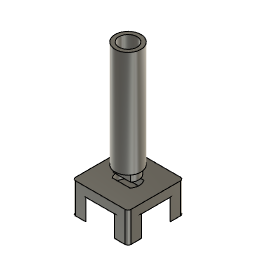
rotating arm cube v4 (Autodesk Fusion 360 design; units mm, degrees)
Autodesk Fusion 360 part; units mm, degrees
note: some values were not read from the file. Set by a fixed rule: which sketch regions a step uses.
sketch "Sketch1" plane through (0, 0, 0) normal (0, 0, 1) x (1, 0, 0)
  line L0 (0, 0) -> (18.3, 0)
  line L1 (18.3, 0) -> (18.3, -18.3)
  line L2 (18.3, -18.3) -> (0, -18.3)
  line L3 (0, -18.3) -> (0, 0)
  circle A0 centre (9.15, -9.15) radius 10.675
  dimension "d1" = 18.3
  dimension "d2" = 18.3
  dimension "d3" = 21.35
  constraint horizontal L0
  constraint vertical L1
  constraint horizontal L2
  constraint vertical L3
  constraint coincident L0.start L3.end
  measures "d1" distance of L0.start L0.end
  measures "d2" distance of L0.start L2.end
  measures "d3" diameter of A0
extrude "Extrude1" add sketch "Sketch1" along normal blind 10 contours L0 L3 A0 | L0 L1 L2 L3 A0 | L0 L1 A0 | L2 L3 A0 | L1 L2 A0 makes body 1
fillet "Fillet1" radius 5.5 4 edges at (18.3, -18.3, 5) (0, -18.3, 5) (18.3, 0, 5) (0, 0, 5) on bodies 1
extrude "Extrude2" add sketch "Sketch1" along normal blind 3 from surface at 10 separate body contours L0 L3 A0 | L0 L1 L2 L3 A0 | L0 L1 A0 | L2 L3 A0 | L1 L2 A0 makes body 2
sketch "Sketch2" plane through (0, 0, 10) normal (0, 0, 1) x (-1, 0, 0)
  arc A0 (-5.5, 0) -> (0, 5.5) centre (-5.5, 5.5) ccw
  line L0 (0, 5.5) -> (0, 12.8)
  arc A1 (0, 12.8) -> (-5.5, 18.3) centre (-5.5, 12.8) ccw
  line L1 (-5.5, 18.3) -> (-12.8, 18.3)
  arc A2 (-12.8, 18.3) -> (-18.3, 12.8) centre (-12.8, 12.8) ccw
  line L2 (-18.3, 12.8) -> (-18.3, 5.5)
  arc A3 (-18.3, 5.5) -> (-12.8, 0) centre (-12.8, 5.5) ccw
  line L3 (-12.8, 0) -> (-5.5, 0)
  line L4 (0, 0) -> (-18.3, 0)
  line L5 (-18.3, 0) -> (-18.3, 18.3)
  line L6 (-18.3, 18.3) -> (0, 18.3)
  line L7 (0, 18.3) -> (0, 0)
  constraint horizontal L4
  constraint vertical L5
  constraint horizontal L6
  constraint vertical L7
  constraint coincident L4.start L7.end
extrude "Extrude3" add sketch "Sketch2" against normal blind 7 contours A0 L4 L7 | A3 L4 L5 | A1 L6 L7 | A2 L5 L6 bodies 2
fillet "Fillet2" radius 1 4 edges at (0, -18.3, 8) (18.3, -18.3, 8) (18.3, 0, 8) (0, 0, 8) on bodies 2
sketch "Sketch3" plane through (0, 0, 13) normal (0, 0, 1) x (-1, 0, 0)
  arc A0 (-1, 0) -> (0, 1) centre (-1, 1) ccw
  line L0 (0, 1) -> (0, 17.3)
  arc A1 (0, 17.3) -> (-1, 18.3) centre (-1, 17.3) ccw
  line L1 (-1, 18.3) -> (-17.3, 18.3)
  arc A2 (-17.3, 18.3) -> (-18.3, 17.3) centre (-17.3, 17.3) ccw
  line L2 (-18.3, 17.3) -> (-18.3, 1)
  arc A3 (-18.3, 1) -> (-17.3, 0) centre (-17.3, 1) ccw
  line L3 (-17.3, 0) -> (-1, 0)
  line L4 (-9.15, 0) -> (-9.15, 18.3) construction
  line L5 (0, 9.15) -> (-18.3, 9.15) construction
  circle A4 centre (-9.15, 9.15) radius 3.5
  line L6 (-8.15, 14.15) -> (-10.15, 14.15)
  line L7 (-10.15, 14.15) -> (-10.15, 4.15)
  line L8 (-10.15, 4.15) -> (-8.15, 4.15)
  line L9 (-8.15, 4.15) -> (-8.15, 14.15)
  line L10 (-8.15, 14.15) -> (-10.15, 4.15) construction
  line L11 (-10.15, 14.15) -> (-8.15, 4.15) construction
  line L12 (-8.05, 4.05) -> (-10.25, 4.05)
  line L13 (-10.25, 4.05) -> (-10.25, 14.25)
  line L14 (-10.25, 14.25) -> (-8.05, 14.25)
  line L15 (-8.05, 14.25) -> (-8.05, 4.05)
  line L16 (-8.05, 4.05) -> (-10.25, 14.25) construction
  line L17 (-10.25, 4.05) -> (-8.05, 14.25) construction
  circle A5 centre (-9.15, 9.15) radius 3.6
  point P0 (-9.15, 9.15)
  point P1 (-9.15, 9.15)
  dimension "d15" = 7
  dimension "d16" = 2
  dimension "d17" = 10
  dimension "d18" = 2.2
  dimension "d19" = 10.2
  dimension "d20" = 7.2
  constraint midpoint L3 L4.start
  constraint midpoint L1 L4.end
  constraint midpoint L0 L5.start
  constraint midpoint L2 L5.end
  constraint midpoint L5 P1
  constraint horizontal L6
  constraint perpendicular L6 L7
  constraint parallel L6 L8
  constraint parallel L7 L9
  constraint coincident L10 P1
  constraint coincident L11 P1
  constraint coincident P1 P0
  constraint horizontal L12
  constraint perpendicular L12 L13
  constraint parallel L12 L14
  constraint parallel L13 L15
  constraint coincident L16 P1
  constraint coincident L17 P1
  measures "d15" diameter of A4
  measures "d16" distance of L7.end L8.end
  measures "d17" distance of L6.end L7.end
  measures "d18" distance of L13.end L14.end
  measures "d19" distance of L12.end L13.end
  measures "d20" diameter of A5
extrude "Extrude5" add sketch "Sketch3" against normal blind 2.5 separate body contours A4 L15 | A4 L9 L15 | A4 L7 L9 | A4 L7 L13 | A4 L13 makes body 3
extrude "Extrude6" add sketch "Sketch3" along normal blind 10 contours A4 L15 | A4 L9 L15 | A4 L7 L9 | A4 L7 L13 | A4 L13 bodies 3
sketch "Sketch5" plane through (0, 0, 10) normal (0, 0, -1) x (1, 0, 0)
  arc A0 (18.3, 12.8) -> (12.8, 18.3) centre (12.8, 12.8) ccw
  line L0 (12.8, 18.3) -> (5.5, 18.3)
  arc A1 (5.5, 18.3) -> (0, 12.8) centre (5.5, 12.8) ccw
  line L1 (0, 12.8) -> (0, 5.5)
  arc A2 (0, 5.5) -> (5.5, 0) centre (5.5, 5.5) ccw
  line L2 (5.5, 0) -> (12.8, 0)
  arc A3 (12.8, 0) -> (18.3, 5.5) centre (12.8, 5.5) ccw
  line L3 (18.3, 5.5) -> (18.3, 12.8)
  line L4 (-0.1, 12.8) -> (-0.1, 5.5)
  arc A4 (-0.1, 5.5) -> (5.5, -0.1) centre (5.5, 5.5) ccw
  line L5 (5.5, -0.1) -> (12.8, -0.1)
  arc A5 (12.8, -0.1) -> (18.4, 5.5) centre (12.8, 5.5) ccw
  line L6 (18.4, 5.5) -> (18.4, 12.8)
  arc A6 (18.4, 12.8) -> (12.8, 18.4) centre (12.8, 12.8) ccw
  line L7 (12.8, 18.4) -> (5.5, 18.4)
  arc A7 (5.5, 18.4) -> (-0.1, 12.8) centre (5.5, 12.8) ccw
  dimension "d33" = 0.1
extrude "Extrude9" cut sketch "Sketch5" along normal blind 7 bodies 2
sketch "Sketch7" plane through (0, 0, 13) normal (0, 0, 1) x (-1, 0, 0)
  arc A0 (-1, 0) -> (0, 1) centre (-1, 1) ccw
  line L0 (0, 1) -> (0, 17.3)
  arc A1 (0, 17.3) -> (-1, 18.3) centre (-1, 17.3) ccw
  line L1 (-1, 18.3) -> (-17.3, 18.3)
  arc A2 (-17.3, 18.3) -> (-18.3, 17.3) centre (-17.3, 17.3) ccw
  line L2 (-18.3, 17.3) -> (-18.3, 1)
  arc A3 (-18.3, 1) -> (-17.3, 0) centre (-17.3, 1) ccw
  line L3 (-17.3, 0) -> (-1, 0)
  line L4 (0, 0) -> (-18.3, 0)
  line L5 (-18.3, 0) -> (-18.3, 18.3)
  line L6 (-18.3, 18.3) -> (0, 18.3)
  line L7 (0, 18.3) -> (0, 0)
  line L8 (0, 0) -> (-18.3, 18.3) construction
  line L9 (0, 18.3) -> (-18.3, 0) construction
  circle A4 centre (-9.15, 9.15) radius 3.7
  line L10 (-5.45, 11.4) -> (-12.85, 11.4)
  line L11 (-12.85, 11.4) -> (-12.85, 6.9)
  line L12 (-12.85, 6.9) -> (-5.45, 6.9)
  line L13 (-5.45, 6.9) -> (-5.45, 11.4)
  line L14 (-5.45, 11.4) -> (-12.85, 6.9) construction
  line L15 (-12.85, 11.4) -> (-5.45, 6.9) construction
  line L16 (-12.85, 7.15) -> (-5.45, 7.15)
  line L17 (-5.45, 7.15) -> (-5.45, 11.15)
  line L18 (-5.45, 11.15) -> (-12.85, 11.15)
  line L19 (-12.85, 11.15) -> (-12.85, 7.15)
  line L20 (-12.85, 7.15) -> (-5.45, 11.15) construction
  line L21 (-5.45, 7.15) -> (-12.85, 11.15) construction
  circle A5 centre (-9.15, 9.15) radius 1
  point P0 (-9.15, 9.15)
  point P1 (-9.15, 9.15)
  dimension "d44" = 18.3
  dimension "d45" = 18.3
  dimension "d46" = 7.4
  dimension "d47" = 7.4
  dimension "d48" = 4.5
  dimension "d49" = 4
  dimension "d60" = 2
  constraint horizontal L4
  constraint vertical L5
  constraint horizontal L6
  constraint vertical L7
  constraint coincident L4.start L7.end
  constraint midpoint L9 P1
  constraint horizontal L10
  constraint perpendicular L10 L11
  constraint parallel L10 L12
  constraint parallel L11 L13
  constraint coincident L14 P1
  constraint coincident L15 P1
  constraint coincident P1 P0
  constraint horizontal L16
  constraint perpendicular L16 L17
  constraint parallel L16 L18
  constraint parallel L17 L19
  constraint coincident L20 P1
  constraint coincident L21 P1
  measures "d44" distance of L4.start L4.end
  measures "d45" distance of L4.start L6.end
  measures "d46" diameter of A4
  measures "d47" distance of L11.end L12.end
  measures "d48" distance of L10.end L11.end
  measures "d49" distance of L16.end L17.end
  measures "d60" diameter of A5
extrude "Extrude11" cut sketch "Sketch7" against normal blind 2.5 contours A4 L16 L18 | A4 L10 L18 | A4 L12 L16 | A5 bodies 2
extrude "Extrude12" cut sketch "Sketch7" against normal blind 10 contours A4 L10 L18 | A4 L12 L16 | A4 L10 | A4 L12 bodies 3
sketch "Sketch8" plane through (0, 0, 23) normal (0, 0, 1) x (-1, 0, 0)
  circle A0 centre (-9.15, 9.15) radius 3.5
  circle A1 centre (-9.15, 9.15) radius 4.25
  circle A2 centre (-9.15, 9.15) radius 3
  dimension "d65" = 8.5
  dimension "d73" = 6
  constraint concentric A1 A2
  measures "d65" diameter of A1
  measures "d73" diameter of A2
extrude "Extrude14" add sketch "Sketch8" against normal blind 9.9 contours A0 | A1 bodies 3
extrude "Extrude15" cut 2 faces at (8.7931, -6.1725, 13) (9.2796, -12.0057, 13) along direction (0, 0, 1) blind 0.1 on bodies 3 bodies 3
extrude "Extrude16" cut sketch "Sketch8" against normal blind 8 contours A2 bodies 3
extrude "Extrude17" add 1 faces at (5.3437, -8.7898, 23) along direction (0, 0, 1) blind 40 on bodies 3 bodies 3
move_body "Move2" bodies 3 to x (1, 0, 0) y (0, 1, 0) z (0, 0, 1) at (0, 0, 4)
ref_plane "WorkPlane3" through (9.15, -4.9, 51.4672) normal (0, 1, 0) x (-1, 0, 0)
extrude "Extrude19" cut 1 faces at (5.3437, -8.7898, 67) along direction (0, 0, -1) blind 14.9 on bodies 3 bodies 3
sketch "Sketch10" plane through (9.15, -4.9, 51.4672) normal (0, 1, 0) x (1, 0, 0)
  line L0 (0, 0) -> (0, -0.63) construction
  line L1 (0, -0.63) -> (0, 4.37) construction
  circle A0 centre (0, 4.37) radius 1.5
  dimension "d93" = 0.63
  dimension "d94" = 5
  dimension "d95" = 3
  constraint coincident L0.start origin
  constraint vertical L0
  constraint parallel L0 L1
  constraint coincident L1.end A0.centre
  measures "d93" distance of L0.start L0.end
  measures "d94" distance of L0.end L1.end
  measures "d95" diameter of A0
extrude "Extrude20" [suppressed]
hidden bodies 1
named bodies: "cube_cap", "cube_arm"
